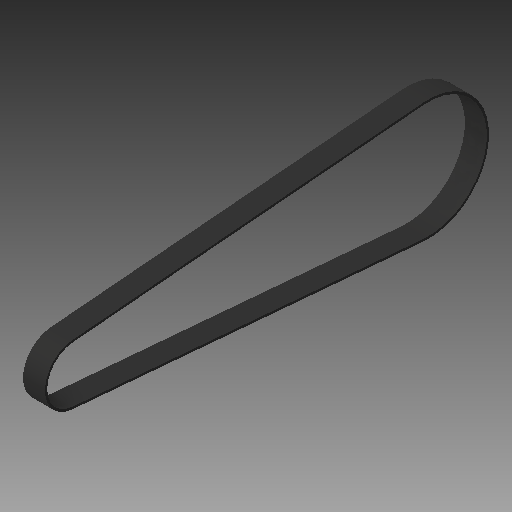
# Autodesk Inventor part: 24 - 50 HTD 134 T Belt
Saved by Autodesk Inventor 2019.4 (Build 234330000, 330)
## iProperties
Created: 2020-01-01
Part Number: 24 - 50 HTD 134 T Belt
Material: Rubber
Document SubType Name: Modeling
Designer: Mark
Mass: 14.1221 g
Surface Area: 222.715 cm^2
Volume: 15.1851 cm^3
Density: 0.93 g/cm^3
Appearance: Rubber - Black
Author: Mark
Autodesk Inventor part; units mm, degrees
ref_plane "YZ Plane" through (0, 0, 0) normal (1, 0, 0) x (0, 1, 0)
ref_plane "XZ Plane" through (0, 0, 0) normal (0, 1, 0) x (-1, 0, 0)
ref_plane "XY Plane" through (0, 0, 0) normal (0, 0, 1) x (1, 0, 0)
sketch "Sketch1" plane through (0, 0, 0) normal (1, 0, 0) x (0, 1, 0)
  arc A0 (19.1, 0) -> (-19.0299, 1.635) centre (0, 0) ccw
  arc A1 (-39.6439, -238.2939) -> (39.6439, -238.2939) centre (0, -241.7) ccw
  line L0 (0, 0) -> (0, -30) construction
  line L1 (0, 0) -> (30, 0) construction
  line L2 (39.6439, -238.2939) -> (19.0299, 1.635)
  line L3 (-19.0299, 1.635) -> (-39.6439, -238.2939)
  arc A2 (20.6, 0) -> (-20.5244, 1.7634) centre (0, 0) ccw
  arc A3 (-41.1384, -238.1655) -> (41.1384, -238.1655) centre (0, -241.7) ccw
  line L4 (41.1384, -238.1655) -> (20.5244, 1.7634)
  line L5 (-41.1384, -238.1655) -> (-20.5244, 1.7634)
  dimension "d0" = 38.2
  dimension "d1" = 79.58
  dimension "d2" = 30
  dimension "d3" = 90
  dimension "d4" = 241.7
  dimension "d5" = 41.2
  dimension "d6" = 82.58
  constraints: 12 end point, 10 point on circle, 8 tangent, 4 centre point, 3 coincident, 3 point on line, 1 horizontal, 1 perpendicular, 1 vertical
  measures "d0" diameter of A0
  measures "d1" diameter of A1
  measures "d2" distance of L0.start L0.end
  measures "d3" angle of L0 L1
  measures "d4" distance of point (0, 0) A1.centre
  measures "d5" diameter of A2
  measures "d6" diameter of A3
extrude "Extrusion1" add sketch "Sketch1" along normal blind 15
body "Solid1"
